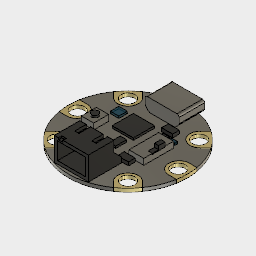
3501 GEMMA M0 (Autodesk Fusion 360 design; units mm, degrees)
Autodesk Fusion 360 part; units mm, degrees
sketch "PCB" plane through (0, 0, 0) normal (0, 0, 1) x (1, 0, 0)
  circle A0 centre (0, 0) radius 14
  circle A1 centre (-11.811, 0) radius 1.59
  circle A2 centre (-8.3516, -8.3516) radius 1.59
  circle A3 centre (8.3516, -8.3516) radius 1.59
  circle A4 centre (11.811, 0) radius 1.59
  circle A5 centre (8.3516, 8.3516) radius 1.59
  circle A6 centre (-8.3516, 8.3516) radius 1.59
  line L0 (-13.7928, -2.4) -> (-12, -2.4)
  arc A7 (-12, -2.4) -> (-12, 2.4) centre (-12, 0) ccw
  line L1 (-12, 2.4) -> (-13.7928, 2.4)
  line L2 (-8.0559, -11.45) -> (-6.7882, -10.1823)
  arc A8 (-6.7882, -10.1823) -> (-10.1823, -6.7882) centre (-8.4853, -8.4853) ccw
  line L3 (-10.1823, -6.7882) -> (-11.45, -8.0559)
  line L4 (11.45, -8.0559) -> (10.1823, -6.7882)
  arc A9 (10.1823, -6.7882) -> (6.7882, -10.1823) centre (8.4853, -8.4853) ccw
  line L5 (6.7882, -10.1823) -> (8.0559, -11.45)
  line L6 (13.7928, 2.4) -> (12, 2.4)
  arc A10 (12, 2.4) -> (12, -2.4) centre (12, 0) ccw
  line L7 (12, -2.4) -> (13.7928, -2.4)
  line L8 (8.0559, 11.45) -> (6.7882, 10.1823)
  arc A11 (6.7882, 10.1823) -> (10.1823, 6.7882) centre (8.4853, 8.4853) ccw
  line L9 (10.1823, 6.7882) -> (11.45, 8.0559)
  line L10 (-11.45, 8.0559) -> (-10.1823, 6.7882)
  arc A12 (-10.1823, 6.7882) -> (-6.7882, 10.1823) centre (-8.4853, 8.4853) ccw
  line L11 (-6.7882, 10.1823) -> (-8.0559, 11.45)
  dimension "d1" = 28
  dimension "d2" = 3.18
  dimension "d3" = 11.811
  dimension "d5" = 360
  dimension "d8" = 4.8
  dimension "d10" = 360
  measures "d1" diameter of A0
  measures "d2" diameter of A1
  measures "d3" distance of A0.centre A1.centre
  measures "d8" diameter of A7
extrude "Extrude1" add sketch "PCB" along normal blind 0.8 makes body 1
extrude "Extrude2" cut sketch "PCB" along normal up to surface (0.8 mm away) contours A0 L6 A10 L7 | A0 L8 A11 L9 | A0 L4 A9 L5 | A0 L10 A12 L11 | A0 L2 A8 L3 | A0 L0 A7 L1 keep common part bodies 1 makes body 2 at (10.5011, -7.5757, 0) makes body 3 at (-10.5011, -7.5757, 0) makes body 4 at (12.7996, 2.059, 0.8) makes body 5 at (-12.7996, 2.059, 0) makes body 6 at (-10.5011, 7.5757, 0)
extrude "Extrude3" add sketch "PCB" along normal blind 0.8 separate body contours A0 L0 A7 L1 L2 A8 L3 L4 A9 L5 L6 A10 L7 L8 A11 L9 L10 A12 L11 makes body 7
ref_plane "WorkPlane1" through (0, 0, 0.8) normal (0, 0, 1) x (1, 0, 0)
sketch "JST connector" plane through (0, 0, 0.8) normal (0, 0, 1) x (1, 0, 0)
  line L0 (-4, -13.3) -> (4, -13.3)
  line L1 (4, -13.3) -> (4, -5.5)
  line L2 (4, -5.5) -> (3.15, -5.5)
  line L3 (3.15, -5.5) -> (3.15, -7.3)
  line L4 (3.15, -7.3) -> (-3.15, -7.3)
  line L5 (-3.15, -7.3) -> (-3.15, -5.5)
  line L6 (-3.15, -5.5) -> (-4, -5.5)
  line L7 (-4, -5.5) -> (-4, -13.3)
  line L8 (0, -13.3) -> (0, -7.3) construction
  line L9 (0, 0) -> (7.5, 0) construction
  line L10 (0, 0) -> (0, 7.5) construction
  line L11 (-4, -7.3) -> (4, -7.3)
  dimension "d16" = 8
  dimension "d17" = 7.8
  dimension "d18" = 0.85
  dimension "d19" = 6
  measures "d16" distance of L0.start L0.end
  measures "d17" distance of L0.start L6.end
  measures "d18" distance of L5.end L6.end
  measures "d19" distance of L0 L4
extrude "Extrude4" add sketch "JST connector" along normal blind 5.5 separate body contours L0 L1 L4 L7 L11 makes body 8
extrude "Extrude5" add sketch "JST connector" along normal blind 3 contours L5 L6 L7 L11 | L1 L2 L3 L11 bodies 8
chamfer "Chamfer1" distance 1.8 angle 45 2 edges at (3.575, -5.5, 3.8) (-3.575, -5.5, 3.8) on bodies 8
shell "Shell1" thickness 0.75 removed faces 1 at (-1.3333, -13.3, 2.6333) on bodies 8
sketch "JST cutter" plane through (0, 0, 6.3) normal (0, 0, 1) x (-1, 0, 0)
  line L0 (4, 13.3) -> (-4, 13.3)
  line L1 (-4, 13.3) -> (-4, 7.3)
  line L2 (-4, 7.3) -> (4, 7.3)
  line L3 (4, 7.3) -> (4, 13.3)
  line L4 (2.5, 7.3) -> (1.5, 7.3)
  line L5 (1.5, 7.3) -> (1.5, 10)
  line L6 (1.5, 10) -> (2.5, 10)
  line L7 (2.5, 10) -> (2.5, 7.3)
  line L8 (0, 7.3) -> (0, 13.3) construction
  line L9 (-2.5, 7.3) -> (-1.5, 7.3)
  line L10 (-1.5, 7.3) -> (-1.5, 10)
  line L11 (-1.5, 10) -> (-2.5, 10)
  line L12 (-2.5, 10) -> (-2.5, 7.3)
  line L13 (3, 12.5) -> (2, 12.5)
  line L14 (2, 12.5) -> (2, 13.3)
  line L15 (2, 13.3) -> (3, 13.3)
  line L16 (3, 13.3) -> (3, 12.5)
  dimension "d26" = 1
  dimension "d27" = 1.5
  measures "d26" distance of L5.end L6.end
  measures "d27" distance of L5 L8
extrude "Extrude6" cut sketch "JST cutter" against normal blind 0.75 contours L2 L4 L5 L6 L7 | L2 L9 L10 L11 L12 bodies 8
extrude "Extrude7" cut sketch "JST cutter" against normal blind 0.4 contours L0 L13 L14 L15 L16 bodies 8
sketch "microUSB" plane through (0, 0, 0.8) normal (0, 0, 1) x (1, 0, 0)
  line L0 (4, 8) -> (-4, 8)
  line L1 (-4, 8) -> (-4, 14)
  line L2 (-4, 14) -> (4, 14)
  line L3 (4, 14) -> (4, 8)
  line L4 (4, 8) -> (-4, 14) construction
  line L5 (-4, 8) -> (4, 14) construction
  line L6 (0, 0) -> (7.5, 0) construction
  point P0 (0, 11)
  dimension "d32" = 6
  dimension "d33" = 8
  dimension "d99" = 11
  measures "d32" distance of L0.end L1.end
  measures "d33" distance of L1.end L2.end
  measures "d99" distance of P0 L6
extrude "Extrude8" add sketch "microUSB" along normal blind 3 separate body makes body 9
chamfer "Chamfer2" distance 1 angle 45 2 edges at (4, 11, 0.8) (-4, 11, 0.8) on bodies 9
fillet "Fillet1" radius 0.5 6 edges at (4, 11, 3.8) (3, 11, 0.8) (4, 11, 1.8) (-3, 11, 0.8) (-4, 11, 1.8) (-4, 11, 3.8) on bodies 9
shell "Shell3" thickness 0.4 removed faces 1 at (0.931, 14, 2.8) on bodies 9
sketch "switch" plane through (0, 0, 0.8) normal (0, 0, 1) x (1, 0, 0)
  line L0 (7.084, -3.373) -> (3.584, -3.373)
  line L1 (3.584, -3.373) -> (3.584, 3.627)
  line L2 (3.584, 3.627) -> (7.084, 3.627)
  line L3 (7.084, 3.627) -> (7.084, -3.373)
  line L4 (7.084, -3.373) -> (3.584, 3.627) construction
  line L5 (3.584, -3.373) -> (7.084, 3.627) construction
  line L6 (0, 0) -> (9, 0) construction
  point P0 (5.334, 0.127)
  dimension "d40" = 7
  dimension "d41" = 3.5
  dimension "d42" = 5.334
  dimension "d43" = 0.127
  measures "d40" distance of L0.end L1.end
  measures "d41" distance of L1.end L2.end
  measures "d42" distance of L6.start P0
  measures "d43" distance of P0 L6
extrude "Extrude9" add sketch "switch" along normal blind 1.4 separate body makes body 10
sketch "actuator" plane through (0, 0, 2.2) normal (0, 0, 1) x (-1, 0, 0)
  line L0 (-7.084, -3.627) -> (-3.584, -3.627)
  line L1 (-3.584, -3.627) -> (-3.584, 3.373)
  line L2 (-3.584, 3.373) -> (-7.084, 3.373)
  line L3 (-7.084, 3.373) -> (-7.084, -3.627)
  line L4 (-3.584, -0.127) -> (-7.084, -0.127) construction
  line L5 (-7.084, -1.627) -> (-6.084, -1.627)
  line L6 (-6.084, -1.627) -> (-6.084, 1.373)
  line L7 (-6.084, 1.373) -> (-7.084, 1.373)
  line L8 (-7.084, 1.373) -> (-7.084, -1.627)
  line L9 (-6.084, -0.127) -> (-7.084, -0.127)
  dimension "d46" = 3
  dimension "d47" = 1
  measures "d46" distance of L5.start L7.end
  measures "d47" distance of L5.start L5.end
extrude "Extrude10" cut sketch "actuator" against normal blind 0.2 contours L3 L5 L6 L8 L9 | L3 L6 L7 L8 L9 bodies 10
extrude "Extrude11" add sketch "actuator" against normal blind 0.2 separate body contours L3 L5 L6 L8 L9 | L3 L6 L7 L8 L9 makes body 11
extrude "Extrude12" add sketch "actuator" along normal blind 0.84 contours L3 L5 L6 L8 L9 bodies 11
sketch "reset button" plane through (0, 0, 0.8) normal (0, 0, 1) x (1, 0, 0)
  line L0 (-5.9795, -2.0675) -> (-8.8795, -2.0675)
  line L1 (-8.8795, -2.0675) -> (-8.8795, 1.4325)
  line L2 (-8.8795, 1.4325) -> (-5.9795, 1.4325)
  line L3 (-5.9795, 1.4325) -> (-5.9795, -2.0675)
  line L4 (-5.9795, -2.0675) -> (-8.8795, 1.4325) construction
  line L5 (-8.8795, -2.0675) -> (-5.9795, 1.4325) construction
  line L6 (0, 0) -> (-10.8122, 0) construction
  circle A0 centre (-7.4295, -0.3175) radius 0.8
  point P0 (-7.4295, -0.3175)
  dimension "d54" = 2.9
  dimension "d55" = 3.5
  dimension "d56" = 0.3175
  dimension "d57" = 7.4295
  dimension "d58" = 1.6
  measures "d54" distance of L1.end L2.end
  measures "d55" distance of L0.end L1.end
  measures "d56" distance of P0 L6
  measures "d57" distance of L6.start A0.centre
  measures "d58" diameter of A0
extrude "Extrude13" add sketch "reset button" along normal blind 1.4 separate body contours L0 L1 L2 L3 | A0 makes body 12
extrude "Extrude14" add sketch "reset button" along normal blind 0.5 from surface at 1.4 separate body contours A0 makes body 13
sketch "SAMD21" plane through (0, 0, 0.8) normal (0, 0, 1) x (1, 0, 0)
  line L0 (0.8, 0.45) -> (-4.2, 0.45)
  line L1 (-4.2, 0.45) -> (-4.2, 5.45)
  line L2 (-4.2, 5.45) -> (0.8, 5.45)
  line L3 (0.8, 5.45) -> (0.8, 0.45)
  line L4 (0.8, 0.45) -> (-4.2, 5.45) construction
  line L5 (-4.2, 0.45) -> (0.8, 5.45) construction
  line L6 (0, 0) -> (2.5, 0) construction
  line L7 (0, 0) -> (0, 2.5) construction
  point P0 (-1.7, 2.95)
  dimension "d64" = 5
  dimension "d65" = 5
  dimension "d66" = 1.7
  dimension "d67" = 2.95
  measures "d64" distance of L0.end L1.end
  measures "d65" distance of L1.end L2.end
  measures "d66" distance of P0 L7
  measures "d67" distance of P0 L6
extrude "Extrude15" add sketch "SAMD21" along normal blind 0.5 separate body makes body 14
sketch "dotstar mini" plane through (0, 0, 0.8) normal (0, 0, 1) x (1, 0, 0)
  line L0 (-5.35, 3.2) -> (-7.35, 3.2)
  line L1 (-7.35, 3.2) -> (-7.35, 5.2)
  line L2 (-7.35, 5.2) -> (-5.35, 5.2)
  line L3 (-5.35, 5.2) -> (-5.35, 3.2)
  line L4 (-5.35, 3.2) -> (-7.35, 5.2) construction
  line L5 (-7.35, 3.2) -> (-5.35, 5.2) construction
  line L6 (0, 0) -> (3, 0) construction
  line L7 (0, 0) -> (0, 2.5) construction
  point P0 (-6.35, 4.2)
  dimension "d70" = 2
  dimension "d71" = 2
  dimension "d72" = 6.35
  dimension "d73" = 4.2
  measures "d70" distance of L1.end L2.end
  measures "d71" distance of L0.end L1.end
  measures "d72" distance of P0 L7
  measures "d73" distance of P0 L6
extrude "Extrude16" add sketch "dotstar mini" along normal blind 0.5 separate body makes body 15
sketch "LED status" plane through (0, 0, 0.8) normal (0, 0, 1) x (1, 0, 0)
  line L0 (6.719, 4.222) -> (5.219, 4.222)
  line L1 (5.219, 4.222) -> (5.219, 4.922)
  line L2 (5.219, 4.922) -> (6.719, 4.922)
  line L3 (6.719, 4.922) -> (6.719, 4.222)
  line L4 (6.719, 4.222) -> (5.219, 4.922) construction
  line L5 (5.219, 4.222) -> (6.719, 4.922) construction
  line L6 (0, 0) -> (2.5, 0) construction
  line L7 (0, 0) -> (0, 2.5) construction
  line L8 (4.819, 4.222) -> (3.319, 4.222)
  line L9 (3.319, 4.222) -> (3.319, 4.922)
  line L10 (3.319, 4.922) -> (4.819, 4.922)
  line L11 (4.819, 4.922) -> (4.819, 4.222)
  point P0 (5.969, 4.572)
  dimension "d76" = 1.5
  dimension "d77" = 0.7
  dimension "d78" = 4.572
  dimension "d79" = 5.969
  dimension "d102" = -1.9
  dimension "d103" = 0
  measures "d76" distance of L1.end L2.end
  measures "d77" distance of L0.end L1.end
  measures "d78" distance of P0 L6
  measures "d79" distance of P0 L7
extrude "Extrude17" add sketch "LED status" along normal blind 0.5 separate body makes body 16 at (6.219, 4.4553, 0.8) makes body 17 at (4.319, 4.4553, 0.8)
sketch "regulator" plane through (0, 0, 0.8) normal (0, 0, 1) x (1, 0, 0)
  line L0 (0.369, -3.2685) -> (-1.131, -3.2685)
  line L1 (-1.131, -3.2685) -> (-1.131, -0.6685)
  line L2 (-1.131, -0.6685) -> (0.369, -0.6685)
  line L3 (0.369, -0.6685) -> (0.369, -3.2685)
  line L4 (0.369, -3.2685) -> (-1.131, -0.6685) construction
  line L5 (-1.131, -3.2685) -> (0.369, -0.6685) construction
  line L6 (0, 0) -> (3, 0) construction
  line L7 (0, 0) -> (0, 3) construction
  point P0 (-0.381, -1.9685)
  dimension "d82" = 2.6
  dimension "d83" = 1.5
  dimension "d84" = 1.9685
  dimension "d88" = 0.381
  measures "d82" distance of L0.end L1.end
  measures "d83" distance of L1.end L2.end
  measures "d84" distance of P0 L6
  measures "d88" distance of P0 L7
extrude "Extrude18" add sketch "regulator" along normal blind 0.5 separate body makes body 18
sketch "rectifier" plane through (0, 0, 0.8) normal (0, 0, 1) x (1, 0, 0)
  line L0 (5.418, -5.299) -> (2.818, -5.299)
  line L1 (2.818, -5.299) -> (2.818, -3.699)
  line L2 (2.818, -3.699) -> (5.418, -3.699)
  line L3 (5.418, -3.699) -> (5.418, -5.299)
  line L4 (5.418, -5.299) -> (2.818, -3.699) construction
  line L5 (2.818, -5.299) -> (5.418, -3.699) construction
  line L6 (0, 0) -> (2.5, 0) construction
  line L7 (0, 0) -> (0, -2.5) construction
  line L8 (4.9195, 5.55) -> (2.3195, 5.55)
  line L9 (2.3195, 5.55) -> (2.3195, 7.15)
  line L10 (2.3195, 7.15) -> (4.9195, 7.15)
  line L11 (4.9195, 7.15) -> (4.9195, 5.55)
  line L12 (4.9195, 5.55) -> (2.3195, 7.15) construction
  line L13 (2.3195, 5.55) -> (4.9195, 7.15) construction
  point P0 (4.118, -4.499)
  point P1 (3.6195, 6.35)
  dimension "d89" = 2.6
  dimension "d90" = 1.6
  dimension "d91" = 4.118
  dimension "d92" = 4.499
  dimension "d95" = 2.6
  dimension "d96" = 1.6
  dimension "d97" = 6.35
  dimension "d98" = 3.6195
  measures "d89" distance of L1.end L2.end
  measures "d90" distance of L0.end L1.end
  measures "d91" distance of P0 L7
  measures "d92" distance of P0 L6
  measures "d95" distance of L9.end L10.end
  measures "d96" distance of L8.end L9.end
  measures "d97" distance of L6 P1
  measures "d98" distance of L7 P1
extrude "Extrude19" add sketch "rectifier" along normal blind 0.8 separate body makes body 19 at (4.5513, -4.7657, 0.8) makes body 20 at (4.0528, 6.6167, 0.8)
named bodies: "GND", "Vout", "3Vo", "D1 / A0", "D0 / A2", "D2 / A1", "PCB", "JST", "microUSB", "DPDT switch", "switch actuator", "reset button", "reset actuator", "samd21", "dotstar mini", "LED status", "regulator", "rectifier A", "rectifier B", "LED resistor"
